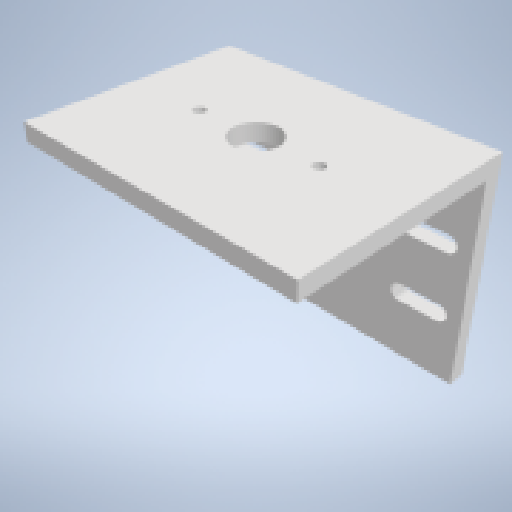
# Autodesk Inventor part: Suporte motor sensor
Saved by Autodesk Inventor 2023 (Build 270158000, 158)
## iProperties
Created: 2022-10-13
Part Number: Suporte motor sensor
Material: Generic
Document SubType Name: Modeling
Designer: klebe
Density: 1 g/cm^3
Appearance: Default
Author: klebe
Autodesk Inventor part; units mm, degrees
ref_plane "YZ Plane" through (0, 0, 0) normal (1, 0, 0) x (0, 1, 0)
ref_plane "XZ Plane" through (0, 0, 0) normal (0, 1, 0) x (-1, 0, 0)
ref_plane "XY Plane" through (0, 0, 0) normal (0, 0, 1) x (1, 0, 0)
sketch "Sketch1" plane through (0, 0, 0) normal (0, 0, 1) x (1, 0, 0)
  line L0 (-200, 100) -> (200, 100) projected
  line L1 (-200, -100) -> (-200, 100) projected
  line L2 (200, -100) -> (-200, -100) projected
  line L3 (121.9, 74) -> (121.9, 71)
  line L4 (171.9, 74) -> (121.9, 74)
  line L5 (171.9, 71) -> (171.9, 35.9)
  line L6 (121.9, 71) -> (171.9, 71)
  line L7 (121.9, 71) -> (121.9, 35.9)
  line L8 (171.9, 35.9) -> (121.9, 35.9)
  line L9 (171.9, 71) -> (171.9, 35.9)
  line L10 (171.9, 74) -> (171.9, 71)
  line L11 (121.9, 35.9) -> (171.9, 35.9)
  line L12 (171.9, 35.9) -> (171.9, 71)
  line L13 (171.9, 71) -> (121.9, 71)
  line L14 (121.9, 71) -> (121.9, 35.9)
  point P0 (0, 0)
  constraints: 24 end point, 2 parallel, 1 horizontal, 1 perpendicular
extrude "Extrusion1" add sketch "Sketch1" along normal blind 3
sketch "Sketch2" plane through (0, 0, 3) normal (0, 0, 1) x (1, 0, 0)
  line L0 (171.9, 74) -> (121.9, 74) projected
  line L1 (171.9, 35.9) -> (171.9, 74) projected
  line L2 (121.9, 74) -> (171.9, 74)
  line L3 (171.9, 74) -> (171.9, 71)
  line L4 (171.9, 71) -> (121.9, 71)
  line L5 (121.9, 71) -> (121.9, 74)
  point P0 (0, 0)
  dimension "d3" = 3
  constraints: 8 end point, 2 parallel, 1 horizontal, 1 perpendicular, 1 point on line
  measures "d3" distance of L2.end L3.end
extrude "Extrusion2" add sketch "Sketch2" along normal blind 35.1
sketch "Sketch3" plane through (121.9, 74, 0) normal (0, 1, 0) x (1, 0, 0)
  line L0 (50, -3) -> (0, -3) projected
  line L1 (50, 0) -> (0, 0) projected
  line L2 (0, 0) -> (0, -38.1) projected
  line L3 (50, -38.1) -> (0, -38.1) projected
  line L4 (50, 0) -> (50, -38.1) projected
  line L5 (50, -3) -> (50, -38.1) projected
  line L6 (36, -19.05) -> (36, -11.2916)
  line L7 (14, -11.2916) -> (14, -19.05)
  line L8 (0, -38.1) -> (0, -19.05)
  line L9 (50, -19.05) -> (60.9839, -19.05)
  point P0 (-121.9, 0)
  point P1 (36, -22.05)
  point P2 (14, -22.05)
  dimension "d25" = 22
  dimension "d33" = 19.05
  constraints: 8 end point, 2 point on line, 1 midpoint, 1 perpendicular
  measures "d25" distance of L6.end L7.start
  measures "d33" distance of L2.end L8.end
sketch "Sketch4" plane through (121.9, 74, 0) normal (0, 1, 0) x (1, 0, 0)
  line L0 (50, 0) -> (0, 0) projected
  line L1 (0, 0) -> (0, -38.1) projected
  line L2 (50, -38.1) -> (0, -38.1) projected
  line L3 (50, 0) -> (50, -38.1) projected
  circle A0 centre (39, -22.05) radius 1 projected
  line L4 (39, -22.05) -> (25, -22.05)
  line L5 (0, -38.1) -> (0, -19.05)
  line L6 (0, -19.05) -> (25, -19.05)
  point P0 (-121.9, 0)
  dimension "d16" = 14
  dimension "d34" = 19.05
  constraints: 6 end point, 1 horizontal, 1 midpoint, 1 perpendicular
  measures "d16" distance of L4.start L4.end
  measures "d34" distance of L1.end L5.end
hole "Hole2" at (146.9, 74, 19.05) direction (0, -1, 0) diameter 8 end through all
hole "Hole3" at (157.9, 74, 19.05) at (135.9, 74, 19.05) direction (0, -1, 0) diameter 2 end through all
sketch "Sketch5" plane through (0, 0, 3) normal (0, 0, 1) x (1, 0, 0)
  line L0 (171.9, 71) -> (121.9, 71) projected
  line L1 (121.9, 71) -> (121.9, 35.9) projected
  line L2 (121.9, 35.9) -> (171.9, 35.9) projected
  line L3 (171.9, 35.9) -> (171.9, 71) projected
  line L4 (166.9, 45.9) -> (167.9, 45.9)
  line L5 (126.9, 45.9) -> (125.9, 45.9)
  line L6 (125.9, 60.9) -> (128.4, 60.9)
  line L7 (167.9, 45.9) -> (160.9, 45.9)
  line L8 (160.9, 48.9) -> (167.9, 48.9)
  line L9 (167.9, 60.9) -> (160.9, 60.9)
  line L10 (160.9, 57.9) -> (167.9, 57.9)
  line L11 (125.9, 60.9) -> (132.9, 60.9)
  line L12 (132.9, 57.9) -> (125.9, 57.9)
  line L13 (125.9, 45.9) -> (132.9, 45.9)
  line L14 (132.9, 48.9) -> (125.9, 48.9)
  arc A0 (167.9, 45.9) -> (167.9, 48.9) centre (167.9, 47.4) ccw
  arc A1 (160.9, 48.9) -> (160.9, 45.9) centre (160.9, 47.4) ccw
  arc A2 (132.9, 45.9) -> (132.9, 48.9) centre (132.9, 47.4) ccw
  arc A3 (125.9, 48.9) -> (125.9, 45.9) centre (125.9, 47.4) ccw
  arc A4 (125.9, 60.9) -> (125.9, 57.9) centre (125.9, 59.4) ccw
  arc A5 (132.9, 57.9) -> (132.9, 60.9) centre (132.9, 59.4) ccw
  arc A6 (160.9, 60.9) -> (160.9, 57.9) centre (160.9, 59.4) ccw
  arc A7 (167.9, 57.9) -> (167.9, 60.9) centre (167.9, 59.4) ccw
  line L15 (132.9, 45.9) -> (126.9, 45.9)
  point P0 (0, 0)
  constraints: 24 end point, 16 point on circle, 13 tangent, 8 centre point, 7 horizontal, 5 parallel
extrude "Extrusion3" cut sketch "Sketch5" against normal blind 3 contours L7 A1 L8 A0 L4 | L5 A3 L14 A2 L13 | L6 L11 A5 L12 A4 | A7 L10 A6 L9
body "Solid1"
